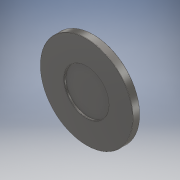
# Autodesk Inventor part: ThrustWasher
Saved by Autodesk Inventor 2018 (Build 220112000, 112)
## iProperties
Created: 2018-04-10
Part Number: ThrustWasher
Material: Steel, Alloy
Document SubType Name: Modeling
Designer: P136265
Density: 7.73 g/cm^3
Appearance: Semi-Polished
Author: P136265
Autodesk Inventor part; units mm, degrees
ref_plane "YZ Plane" through (0, 0, 0) normal (1, 0, 0) x (0, 1, 0)
ref_plane "XZ Plane" through (0, 0, 0) normal (0, 1, 0) x (-1, 0, 0)
ref_plane "XY Plane" through (0, 0, 0) normal (0, 0, 1) x (1, 0, 0)
sketch "Sketch1" plane through (0, 0, 0) normal (0, 1, 0) x (-1, 0, 0)
  circle A0 centre (0, 0) radius 13
  dimension "d0" = 26
  constraints: 1 centre point, 1 coincident
  measures "d0" diameter of A0
extrude "Extrusion1" add sketch "Sketch1" along normal blind 2
sketch "Sketch2" plane through (0, 2, 0) normal (0, 1, 0) x (1, 0, 0)
  circle A0 centre (0, 0) radius 13 construction
  circle A1 centre (0, 0) radius 10.5
  circle A2 centre (0, 0) radius 6.5
  dimension "d3" = 2.5
  dimension "d4" = 4
  constraints: 2 centre point
  measures "d3" radial gap between concentric circles of A0 A1
  measures "d4" radial gap between concentric circles of A1 A2
extrude "Extrusion2" cut sketch "Sketch2" against normal blind 0.3
sketch "Sketch3" plane through (0, 0, 0) normal (0, -1, 0) x (1, 0, 0)
  circle A0 centre (0, 0) radius 6.25
  dimension "d7" = 12.5
  constraints: 1 centre point, 1 coincident
  measures "d7" diameter of A0
extrude "Extrusion3" cut sketch "Sketch3" against normal blind 0.5
fillet "Fillet1" radius 0.1 5 edges at (13, 2, 0) (-10.5, 2, 0) (-6.5, 2, 0) (13, 0, 0) (-6.25, 0, 0)
body "Solid1"
